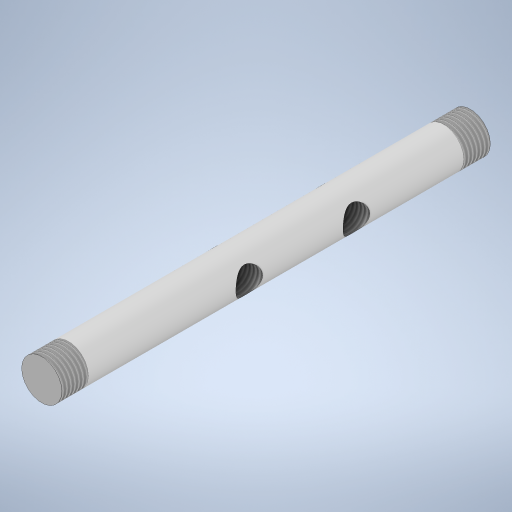
# Autodesk Inventor part: shaft2
Saved by Autodesk Inventor 2023 (Build 270158000, 158)
## iProperties
Created: 2023-07-26
Part Number: shaft2
Material: Generic
Document SubType Name: Modeling
Designer: User
Density: 1 g/cm^3
Appearance: Default
Author: User
Autodesk Inventor part; units mm, degrees
ref_plane "XZ Plane" through (0, 0, 0) normal (0, 1, 0) x (-1, 0, 0)
ref_plane "XY Plane" through (0, 0, 0) normal (0, 0, 1) x (1, 0, 0)
sketch "Sketch1" plane through (0, 0, 0) normal (0, 0, 1) x (1, 0, 0)
  circle A0 centre (0, 0) radius 7.5
  dimension "d0" = 15
  constraints: 1 centre point, 1 coincident
  measures "d0" diameter of A0
extrude "Extrusion1" add sketch "Sketch1" along normal blind 160
ref_plane "Work Plane1" through (7.5, 0, 0) normal (1, 0, 0) x (0, 1, 0)
sketch "Sketch2" plane through (7.5, 0, 0) normal (1, 0, 0) x (0, 1, 0)
  circle A0 centre (0, 50) radius 5
  circle A1 centre (0, 90) radius 5
  line L0 (7.5, 160) -> (-7.5, 160) projected
  point P0 (0, 0)
  dimension "d3" = 10
  dimension "d4" = 10
  dimension "d5" = 40
  dimension "d6" = 70
  constraints: 2 centre point
  measures "d3" diameter of A0
  measures "d4" diameter of A1
  measures "d5" distance of A1.centre A0.centre
  measures "d6" distance from line of A1.centre L0
extrude "Extrusion2" cut sketch "Sketch2" against normal blind 15 contours A0
extrude "Extrusion3" cut sketch "Sketch2" against normal blind 15 contours A1
thread "Thread1" size "M15x1.5" class "6g" standard "ANSI Metric M Profile" length 10
thread "Thread2" size "M15x1.5" class "6g" standard "ANSI Metric M Profile" length 10
thread "Thread3" size "M10x1.5" class "6H" standard "ANSI Metric M Profile" length 10
thread "Thread4" size "M10x1.5" class "6H" standard "ANSI Metric M Profile" length 10
body "Solid1"
